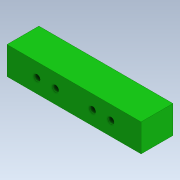
# Autodesk Inventor part: Motor Spacer
Saved by Autodesk Inventor 2020 (Build 240168000, 168)
## iProperties
Created: 2023-01-07
Part Number: Motor Spacer
Material: Generic
Document SubType Name: Modeling
Designer: Allan
Density: 1 g/cm^3
Appearance: Dark Green
Author: Allan
Autodesk Inventor part; units mm, degrees
ref_plane "YZ Plane" through (0, 0, 0) normal (1, 0, 0) x (0, 1, 0)
ref_plane "XZ Plane" through (0, 0, 0) normal (0, 1, 0) x (-1, 0, 0)
ref_plane "XY Plane" through (0, 0, 0) normal (0, 0, 1) x (1, 0, 0)
sketch "Sketch1" plane through (0, 0, 0) normal (0, 0, 1) x (1, 0, 0)
  circle A0 centre (13, 6) radius 1.3525
  circle A1 centre (21, 6) radius 1.3525
  circle A2 centre (37, 6) radius 1.3525
  circle A3 centre (45, 6) radius 1.3525
  line L0 (0, 0) -> (58, 0)
  line L1 (58, 0) -> (58, 12)
  line L2 (0, 12) -> (58, 12)
  line L3 (0, 12) -> (0, 0)
  point P0 (29, 6)
  constraints: 8 end point, 4 centre point
extrude "Extrusion1" add sketch "Sketch1" along normal blind 13.7922
body "Solid1"
